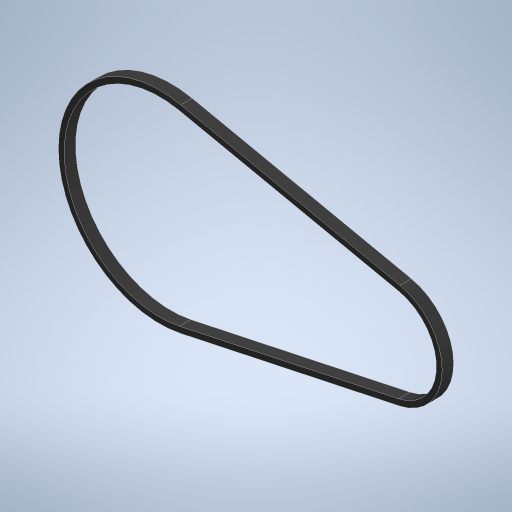
# Autodesk Inventor part: NHK_t0_4
Saved by Autodesk Inventor 2023 (Build 270158000, 158)
## iProperties
Created: 2022-04-19
Part Number: NHK_t0_4
Material: ゴム
Document SubType Name: Modeling
Designer: yuta
Density: 0.93 g/cm^3
Appearance: ゴム - 黒
Author: yuta
Autodesk Inventor part; units mm, degrees
ref_plane "YZ Plane" through (0, 0, 0) normal (1, 0, 0) x (0, 1, 0)
ref_plane "XZ Plane" through (0, 0, 0) normal (0, 1, 0) x (-1, 0, 0)
ref_plane "XY Plane" through (0, 0, 0) normal (0, 0, 1) x (1, 0, 0)
sketch "スケッチ1" plane through (0, 0, 0) normal (0, 0, 1) x (1, 0, 0)
  arc A0 (11.0417, 51.8371) -> (11.0417, -51.8371) centre (0, 0) ccw
  arc A1 (125.8333, -27.3856) -> (125.8333, 27.3856) centre (120, 0) ccw
  line L0 (11.0417, 51.8371) -> (125.8333, 27.3856)
  line L1 (11.0417, -51.8371) -> (125.8333, -27.3856)
  arc A2 (10.4167, 48.9029) -> (10.4167, -48.9029) centre (0, 0) ccw
  arc A3 (125.2083, -24.4514) -> (125.2083, 24.4514) centre (120, 0) ccw
  line L2 (10.4167, 48.9029) -> (125.2083, 24.4514)
  line L3 (10.4167, -48.9029) -> (125.2083, -24.4514)
  point P0 (120, -28)
  point P1 (120, 28)
  dimension "d0" = 106
  dimension "d1" = 56
  dimension "d2" = 120
  dimension "d3" = 28
  dimension "d4" = 100
  dimension "d5" = 50
  constraints: 10 point on circle, 8 end point, 8 tangent, 4 centre point, 3 coincident
  measures "d0" diameter of A0
  measures "d1" diameter of A1
  measures "d2" distance of A1.centre point (0, 0)
  measures "d3" distance of A1.centre point (120, 28)
  measures "d4" diameter of A2
  measures "d5" diameter of A3
extrude "押し出し1" add sketch "スケッチ1" along normal blind 6
